Autodesk Inventor part; units mm, degrees
(part 3 of 3)
  line L339 (-12.89, 134.4688) -> (-12.89, 147.4688)
  line L340 (-26.39, 133.9688) -> (-13.39, 133.9688)
  line L341 (-26.39, 147.9688) -> (-13.39, 147.9688)
  arc A336 (-26.89, 134.4688) -> (-26.39, 133.9688) centre (-26.39, 134.4688) ccw
  arc A337 (-26.39, 147.9688) -> (-26.89, 147.4688) centre (-26.39, 147.4688) ccw
  arc A338 (-13.39, 133.9688) -> (-12.89, 134.4688) centre (-13.39, 134.4688) ccw
  arc A339 (-12.89, 147.4688) -> (-13.39, 147.9688) centre (-13.39, 147.4688) ccw
  line L342 (-25.89, 87.9688) -> (-25.89, 93.9688)
  line L343 (-10.89, 87.9688) -> (-10.89, 93.9688)
  line L344 (-25.39, 87.4688) -> (-11.39, 87.4688)
  line L345 (-25.39, 94.4688) -> (-11.39, 94.4688)
  arc A340 (-25.89, 87.9688) -> (-25.39, 87.4688) centre (-25.39, 87.9688) ccw
  arc A341 (-25.39, 94.4688) -> (-25.89, 93.9688) centre (-25.39, 93.9688) ccw
  arc A342 (-11.39, 87.4688) -> (-10.89, 87.9688) centre (-11.39, 87.9688) ccw
  arc A343 (-10.89, 93.9688) -> (-11.39, 94.4688) centre (-11.39, 93.9688) ccw
  line L346 (-25.89, 187.9688) -> (-25.89, 193.9688)
  line L347 (-10.89, 187.9688) -> (-10.89, 193.9688)
  line L348 (-25.39, 187.4688) -> (-11.39, 187.4688)
  line L349 (-25.39, 194.4688) -> (-11.39, 194.4688)
  arc A344 (-25.89, 187.9688) -> (-25.39, 187.4688) centre (-25.39, 187.9688) ccw
  arc A345 (-25.39, 194.4688) -> (-25.89, 193.9688) centre (-25.39, 193.9688) ccw
  arc A346 (-11.39, 187.4688) -> (-10.89, 187.9688) centre (-11.39, 187.9688) ccw
  arc A347 (-10.89, 193.9688) -> (-11.39, 194.4688) centre (-11.39, 193.9688) ccw
  line L350 (-26.89, 205.9063) -> (-26.89, 218.9063)
  line L351 (-12.89, 205.9063) -> (-12.89, 218.9063)
  line L352 (-26.39, 205.4063) -> (-13.39, 205.4063)
  line L353 (-26.39, 219.4063) -> (-13.39, 219.4063)
  arc A348 (-26.89, 205.9063) -> (-26.39, 205.4063) centre (-26.39, 205.9063) ccw
  arc A349 (-26.39, 219.4063) -> (-26.89, 218.9063) centre (-26.39, 218.9063) ccw
  arc A350 (-13.39, 205.4063) -> (-12.89, 205.9063) centre (-13.39, 205.9063) ccw
  arc A351 (-12.89, 218.9063) -> (-13.39, 219.4063) centre (-13.39, 218.9063) ccw
  line L354 (-26.89, 229.7188) -> (-26.89, 242.7188)
  line L355 (-12.89, 229.7188) -> (-12.89, 242.7188)
  line L356 (-26.39, 229.2188) -> (-13.39, 229.2188)
  line L357 (-26.39, 243.2188) -> (-13.39, 243.2188)
  arc A352 (-26.89, 229.7188) -> (-26.39, 229.2188) centre (-26.39, 229.7188) ccw
  arc A353 (-26.39, 243.2188) -> (-26.89, 242.7188) centre (-26.39, 242.7188) ccw
  arc A354 (-13.39, 229.2188) -> (-12.89, 229.7188) centre (-13.39, 229.7188) ccw
  arc A355 (-12.89, 242.7188) -> (-13.39, 243.2188) centre (-13.39, 242.7188) ccw
  line L358 (-26.89, 253.5313) -> (-26.89, 266.5313)
  line L359 (-12.89, 253.5313) -> (-12.89, 266.5313)
  line L360 (-26.39, 253.0313) -> (-13.39, 253.0313)
  line L361 (-26.39, 267.0313) -> (-13.39, 267.0313)
  arc A356 (-26.89, 253.5313) -> (-26.39, 253.0313) centre (-26.39, 253.5313) ccw
  arc A357 (-26.39, 267.0313) -> (-26.89, 266.5313) centre (-26.39, 266.5313) ccw
  arc A358 (-13.39, 253.0313) -> (-12.89, 253.5313) centre (-13.39, 253.5313) ccw
  arc A359 (-12.89, 266.5313) -> (-13.39, 267.0313) centre (-13.39, 266.5313) ccw
  line L362 (-26.89, 277.3438) -> (-26.89, 290.3438)
  line L363 (-12.89, 277.3438) -> (-12.89, 290.3438)
  line L364 (-26.39, 276.8438) -> (-13.39, 276.8438)
  line L365 (-26.39, 290.8438) -> (-13.39, 290.8438)
  arc A360 (-26.89, 277.3438) -> (-26.39, 276.8438) centre (-26.39, 277.3438) ccw
  arc A361 (-26.39, 290.8438) -> (-26.89, 290.3438) centre (-26.39, 290.3438) ccw
  arc A362 (-13.39, 276.8438) -> (-12.89, 277.3438) centre (-13.39, 277.3438) ccw
  arc A363 (-12.89, 290.3438) -> (-13.39, 290.8438) centre (-13.39, 290.3438) ccw
  line L366 (-26.89, 303.5375) -> (-26.89, 316.5375)
  line L367 (-12.89, 303.5375) -> (-12.89, 316.5375)
  line L368 (-26.39, 303.0375) -> (-13.39, 303.0375)
  line L369 (-26.39, 317.0375) -> (-13.39, 317.0375)
  arc A364 (-26.89, 303.5375) -> (-26.39, 303.0375) centre (-26.39, 303.5375) ccw
  arc A365 (-26.39, 317.0375) -> (-26.89, 316.5375) centre (-26.39, 316.5375) ccw
  arc A366 (-13.39, 303.0375) -> (-12.89, 303.5375) centre (-13.39, 303.5375) ccw
  arc A367 (-12.89, 316.5375) -> (-13.39, 317.0375) centre (-13.39, 316.5375) ccw
  line L370 (-26.89, 322.5875) -> (-26.89, 335.5875)
  line L371 (-12.89, 322.5875) -> (-12.89, 335.5875)
  line L372 (-26.39, 322.0875) -> (-13.39, 322.0875)
  line L373 (-26.39, 336.0875) -> (-13.39, 336.0875)
  arc A368 (-26.89, 322.5875) -> (-26.39, 322.0875) centre (-26.39, 322.5875) ccw
  arc A369 (-26.39, 336.0875) -> (-26.89, 335.5875) centre (-26.39, 335.5875) ccw
  arc A370 (-13.39, 322.0875) -> (-12.89, 322.5875) centre (-13.39, 322.5875) ccw
  arc A371 (-12.89, 335.5875) -> (-13.39, 336.0875) centre (-13.39, 335.5875) ccw
  line L374 (-26.89, 341.6375) -> (-26.89, 354.6375)
  line L375 (-12.89, 341.6375) -> (-12.89, 354.6375)
  line L376 (-26.39, 341.1375) -> (-13.39, 341.1375)
  line L377 (-26.39, 355.1375) -> (-13.39, 355.1375)
  arc A372 (-26.89, 341.6375) -> (-26.39, 341.1375) centre (-26.39, 341.6375) ccw
  arc A373 (-26.39, 355.1375) -> (-26.89, 354.6375) centre (-26.39, 354.6375) ccw
  arc A374 (-13.39, 341.1375) -> (-12.89, 341.6375) centre (-13.39, 341.6375) ccw
  arc A375 (-12.89, 354.6375) -> (-13.39, 355.1375) centre (-13.39, 354.6375) ccw
  line L378 (-10.365, 10) -> (-10.365, 357.6625)
  line L379 (-134.19, 10) -> (-134.19, 357.6625)
  line L380 (-10.365, 10) -> (-134.19, 10)
  line L381 (-10.365, 357.6625) -> (-134.19, 357.6625)
  point P0 (-64.49, 19.6687)
  point P1 (-50.99, 33.1688)
  point P2 (-51.49, 33.6688)
  point P3 (-64.99, 33.1688)
  point P4 (-64.99, 20.1688)
  point P5 (-51.49, 45.8625)
  point P6 (-50.99, 46.3625)
  point P7 (-50.99, 59.3625)
  point P8 (-51.49, 59.8625)
  point P9 (-64.99, 59.3625)
  point P10 (-64.99, 46.3625)
  point P11 (-64.49, 83.9625)
  point P12 (-50.99, 84.4625)
  point P13 (-50.99, 97.4625)
  point P14 (-64.49, 97.9625)
  point P15 (-64.99, 84.4625)
  point P16 (-84.04, 79.7)
  point P17 (-83.54, 79.2)
  point P18 (-70.04, 92.7)
  point P19 (-70.54, 93.2)
  point P20 (-83.54, 93.2)
  point P21 (-84.04, 92.7)
  point P22 (-83.54, 17.2875)
  point P23 (-70.54, 17.2875)
  point P24 (-70.04, 17.7875)
  point P25 (-70.04, 30.7875)
  point P26 (-70.54, 31.2875)
  point P27 (-83.54, 31.2875)
  point P28 (-84.04, 30.7875)
  point P29 (-84.04, 17.7875)
  point P30 (-83.54, 41.1)
  point P31 (-70.54, 41.1)
  point P32 (-70.04, 41.6)
  point P33 (-70.54, 55.1)
  point P34 (-83.54, 55.1)
  point P35 (-84.04, 54.6)
  point P36 (-84.04, 41.6)
  point P37 (-26.89, 39.2188)
  point P38 (-26.39, 38.7188)
  point P39 (-13.39, 38.7188)
  point P40 (-12.89, 39.2188)
  point P41 (-12.89, 52.2188)
  point P42 (-13.39, 52.7188)
  point P43 (-26.39, 52.7188)
  point P44 (-26.89, 52.2188)
  point P45 (-26.39, 62.5313)
  point P46 (-13.39, 62.5313)
  point P47 (-12.89, 76.0313)
  point P48 (-26.89, 63.0313)
  point P49 (-64.49, 64.9125)
  point P50 (-51.49, 64.9125)
  point P51 (-50.99, 65.4125)
  point P52 (-50.99, 78.4125)
  point P53 (-51.49, 78.9125)
  point P54 (-64.49, 78.9125)
  point P55 (-64.99, 78.4125)
  point P56 (-64.99, 65.4125)
  point P57 (-25.39, 87.4688)
  point P58 (-11.39, 87.4688)
  point P59 (-10.89, 87.9688)
  point P60 (-10.89, 93.9688)
  point P61 (-25.39, 94.4688)
  point P62 (-25.89, 93.9688)
  point P63 (-25.89, 87.9688)
  point P64 (-26.39, 14.9063)
  point P65 (-13.39, 14.9063)
  point P66 (-12.89, 15.4063)
  point P67 (-12.89, 28.4063)
  point P68 (-26.39, 28.9063)
  point P69 (-26.89, 28.4063)
  point P70 (-26.89, 15.4063)
  point P71 (-45.44, 24.4313)
  point P72 (-32.44, 24.4313)
  point P73 (-31.94, 24.9313)
  point P74 (-31.94, 37.9313)
  point P75 (-32.44, 38.4313)
  point P76 (-45.44, 38.4313)
  point P77 (-44.44, 15.9933)
  point P78 (-30.44, 15.9933)
  point P79 (-29.94, 16.4933)
  point P80 (-29.94, 22.4933)
  point P81 (-30.44, 22.9933)
  point P82 (-44.94, 22.4933)
  point P83 (-44.44, 39.8693)
  point P84 (-30.44, 39.8693)
  point P85 (-29.94, 46.3692)
  point P86 (-44.44, 46.8693)
  point P87 (-44.94, 46.3693)
  point P88 (-44.94, 40.3693)
  point P89 (-45.44, 55.3875)
  point P90 (-32.44, 55.3875)
  point P91 (-45.44, 69.3875)
  point P92 (-45.94, 68.8875)
  point P93 (-45.94, 55.8875)
  point P94 (-32.44, 74.4375)
  point P95 (-31.94, 87.9375)
  point P96 (-45.44, 88.4375)
  point P97 (-45.94, 87.9375)
  point P98 (-45.94, 74.9375)
  point P99 (-102.59, 12.525)
  point P100 (-89.59, 12.525)
  point P101 (-89.09, 13.025)
  point P102 (-89.09, 26.025)
  point P103 (-89.59, 26.525)
  point P104 (-102.59, 26.525)
  point P105 (-103.09, 26.025)
  point P106 (-103.09, 13.025)
  point P107 (-102.59, 31.575)
  point P108 (-89.09, 32.075)
  point P109 (-89.09, 45.075)
  point P110 (-89.59, 45.575)
  point P111 (-102.59, 45.575)
  point P112 (-103.09, 45.075)
  point P113 (-102.59, 50.625)
  point P114 (-89.59, 50.625)
  point P115 (-89.09, 51.125)
  point P116 (-89.09, 64.125)
  point P117 (-89.59, 64.625)
  point P118 (-102.59, 64.625)
  point P119 (-103.09, 51.125)
  point P120 (-102.59, 69.675)
  point P121 (-89.59, 69.675)
  point P122 (-89.09, 83.175)
  point P123 (-89.59, 83.675)
  point P124 (-103.09, 83.175)
  point P125 (-103.09, 70.175)
  point P126 (-83.54, 60.15)
  point P127 (-70.54, 60.15)
  point P128 (-70.04, 60.65)
  point P129 (-70.54, 74.15)
  point P130 (-84.04, 73.65)
  point P131 (-84.04, 60.65)
  point P132 (-102.59, 88.725)
  point P133 (-89.59, 88.725)
  point P134 (-89.09, 89.225)
  point P135 (-89.09, 102.225)
  point P136 (-89.59, 102.725)
  point P137 (-103.09, 102.225)
  point P138 (-103.09, 89.225)
  point P139 (-131.665, 13.025)
  point P140 (-118.165, 12.525)
  point P141 (-117.665, 13.025)
  point P142 (-117.665, 26.025)
  point P143 (-118.165, 26.525)
  point P144 (-131.165, 26.525)
  point P145 (-131.665, 26.025)
  point P146 (-118.165, 50.625)
  point P147 (-117.665, 64.125)
  point P148 (-118.165, 64.625)
  point P149 (-131.665, 64.125)
  point P150 (-117.665, 83.175)
  point P151 (-131.165, 83.675)
  point P152 (-131.665, 83.175)
  point P153 (-131.665, 70.175)
  point P154 (-131.165, 88.725)
  point P155 (-118.165, 88.725)
  point P156 (-117.665, 89.225)
  point P157 (-117.665, 102.225)
  point P158 (-51.49, 103.0125)
  point P159 (-50.99, 103.5125)
  point P160 (-50.99, 116.5125)
  point P161 (-51.49, 117.0125)
  point P162 (-64.49, 117.0125)
  point P163 (-64.99, 103.5125)
  point P164 (-64.49, 122.0625)
  point P165 (-51.49, 122.0625)
  point P166 (-50.99, 122.5625)
  point P167 (-50.99, 135.5625)
  point P168 (-51.49, 136.0625)
  point P169 (-50.99, 141.6125)
  point P170 (-50.99, 154.6125)
  point P171 (-51.49, 155.1125)
  point P172 (-64.99, 154.6125)
  point P173 (-50.99, 160.6625)
  point P174 (-50.99, 173.6625)
  point P175 (-51.49, 174.1625)
  point P176 (-64.99, 173.6625)
  point P177 (-64.99, 160.6625)
  point P178 (-70.54, 112.25)
  point P179 (-83.54, 112.25)
  point P180 (-84.04, 111.75)
  point P181 (-84.04, 98.75)
  point P182 (-83.54, 117.3)
  point P183 (-70.04, 117.8)
  point P184 (-84.04, 130.8)
  point P185 (-84.04, 117.8)
  point P186 (-83.54, 136.35)
  point P187 (-84.04, 149.85)
  point P188 (-84.04, 136.85)
  point P189 (-83.54, 155.4)
  point P190 (-70.54, 155.4)
  point P191 (-70.04, 155.9)
  point P192 (-70.04, 168.9)
  point P193 (-70.54, 169.4)
  point P194 (-83.54, 169.4)
  point P195 (-84.04, 168.9)
  point P196 (-83.54, 174.45)
  point P197 (-70.54, 174.45)
  point P198 (-70.04, 174.95)
  point P199 (-70.54, 188.45)
  dimension "d67" = 10
  dimension "d68" = 10
extrude "Extrusion2" cut sketch "Sketch3" against normal blind 2 contours L2 A1 L5 A3 L3 A2 L4 A0 | L6 A5 L9 A7 L7 A6 L8 A4 | L10 A9 L13 A11 L11 A10 L12 A8 | L14 A13 L17 A15 L15 A14 L16 A12 | L18 A17 L21 A19 L19 A18 L20 A16 | L22 A21 L25 A23 L23 A22 L24 A20 | L26 A25 L29 A27 L27 A26 L28 A24 | L30 A29 L33 A31 L31 A30 L32 A28 | L34 A33 L37 A35 L35 A34 L36 A32 | L38 A37 L41 A39 L39 A38 L40 A36 | L42 A41 L45 A43 L43 A42 L44 A40 | L46 A45 L49 A47 L47 A46 L48 A44 | L50 A49 L53 A51 L51 A50 L52 A48 | L54 A53 L57 A55 L55 A54 L56 A52 | L58 A57 L61 A59 L59 A58 L60 A56 | L62 A61 L65 A63 L63 A62 L64 A60 | L66 A65 L69 A67 L67 A66 L68 A64 | L70 A69 L73 A71 L71 A70 L72 A68 | L74 A73 L77 A75 L75 A74 L76 A72 | L78 A77 L81 A79 L79 A78 L80 A76 | L82 A81 L85 A83 L83 A82 L84 A80 | L86 A85 L89 A87 L87 A86 L88 A84 | L90 A89 L93 A91 L91 A90 L92 A88 | L94 A93 L97 A95 L95 A94 L96 A92 | L98 A97 L101 A99 L99 A98 L100 A96 | L102 A101 L105 A103 L103 A102 L104 A100 | L106 A105 L109 A107 L107 A106 L108 A104 | L110 A109 L113 A111 L111 A110 L112 A108 | L114 A113 L117 A115 L115 A114 L116 A112 | L118 A117 L121 A119 L119 A118 L120 A116 | L122 A121 L125 A123 L123 A122 L124 A120 | L126 A125 L129 A127 L127 A126 L128 A124 | L130 A129 L133 A131 L131 A130 L132 A128 | L134 A133 L137 A135 L135 A134 L136 A132 | L138 A137 L141 A139 L139 A138 L140 A136 | L142 A141 L145 A143 L143 A142 L144 A140 | L146 A145 L149 A147 L147 A146 L148 A144 | L150 A149 L153 A151 L151 A150 L152 A148 | L154 A153 L157 A155 L155 A154 L156 A152 | L158 A157 L161 A159 L159 A158 L160 A156 | L162 A161 L165 A163 L163 A162 L164 A160 | L166 A165 L169 A167 L167 A166 L168 A164 | L170 A169 L173 A171 L171 A170 L172 A168 | L174 A173 L177 A175 L175 A174 L176 A172 | L178 A177 L181 A179 L179 A178 L180 A176 | L182 A181 L185 A183 L183 A182 L184 A180 | L186 A185 L189 A187 L187 A186 L188 A184 | L190 A189 L193 A191 L191 A190 L192 A188 | L194 A193 L197 A195 L195 A194 L196 A192 | L198 A197 L201 A199 L199 A198 L200 A196 | L202 A201 L205 A203 L203 A202 L204 A200 | L206 A205 L209 A207 L207 A206 L208 A204 | L210 A209 L213 A211 L211 A210 L212 A208 | L214 A213 L217 A215 L215 A214 L216 A212 | L218 A217 L221 A219 L219 A218 L220 A216 | L222 A221 L225 A223 L223 A222 L224 A220 | L226 A225 L229 A227 L227 A226 L228 A224 | L230 A229 L233 A231 L231 A230 L232 A228 | L234 A233 L237 A235 L235 A234 L236 A232 | L238 A237 L241 A239 L239 A238 L240 A236 | L242 A241 L245 A243 L243 A242 L244 A240 | L246 A245 L249 A247 L247 A246 L248 A244 | L250 A249 L253 A251 L251 A250 L252 A248 | L254 A253 L257 A255 L255 A254 L256 A252 | L258 A257 L261 A259 L259 A258 L260 A256 | L262 A261 L265 A263 L263 A262 L264 A260 | L266 A265 L269 A267 L267 A266 L268 A264 | L270 A269 L273 A271 L271 A270 L272 A268 | L274 A273 L277 A275 L275 A274 L276 A272 | L278 A277 L281 A279 L279 A278 L280 A276 | L282 A281 L285 A283 L283 A282 L284 A280 | L286 A285 L289 A287 L287 A286 L288 A284 | L290 A289 L293 A291 L291 A290 L292 A288 | L294 A293 L297 A295 L295 A294 L296 A292 | L298 A297 L301 A299 L299 A298 L300 A296 | L302 A301 L305 A303 L303 A302 L304 A300 | L306 A305 L309 A307 L307 A306 L308 A304 | L310 A309 L313 A311 L311 A310 L312 A308 | L314 A313 L317 A315 L315 A314 L316 A312 | L318 A317 L321 A319 L319 A318 L320 A316 | L322 A321 L325 A323 L323 A322 L324 A320 | L326 A325 L329 A327 L327 A326 L328 A324 | L330 A329 L333 A331 L331 A330 L332 A328 | L334 A333 L337 A335 L335 A334 L336 A332 | L338 A337 L341 A339 L339 A338 L340 A336 | L342 A341 L345 A343 L343 A342 L344 A340 | L346 A345 L349 A347 L347 A346 L348 A344 | L350 A349 L353 A351 L351 A350 L352 A348 | L354 A353 L357 A355 L355 A354 L356 A352 | L358 A357 L361 A359 L359 A358 L360 A356 | L362 A361 L365 A363 L363 A362 L364 A360 | L366 A365 L369 A367 L367 A366 L368 A364 | L370 A369 L373 A371 L371 A370 L372 A368 | L374 A373 L377 A375 L375 A374 L376 A372
body "Solid1"
